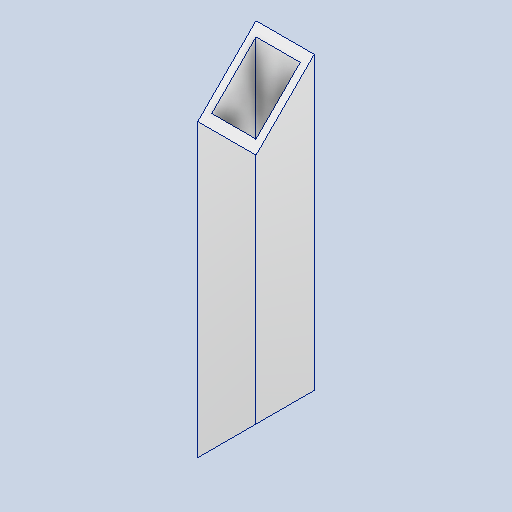
# Autodesk Inventor part: P407
Saved by Autodesk Inventor 2023 (Build 270158000, 158)
## iProperties
Created: 2022-08-29
Part Number: P407
Material: Aluminum 6061
Document SubType Name: Modeling
Designer: D.C. Eksteen
Density: 2.7 g/cm^3
Appearance: Aluminum - Flat
Author: D.C. Eksteen
Title: FRONT PLATFORM TUBE
Autodesk Inventor part; units mm, degrees
ref_plane "YZ Plane" through (0, 0, 0) normal (1, 0, 0) x (0, 1, 0)
ref_plane "XZ Plane" through (0, 0, 0) normal (0, 1, 0) x (-1, 0, 0)
ref_plane "XY Plane" through (0, 0, 0) normal (0, 0, 1) x (1, 0, 0)
sketch "Sketch1" plane through (0, 0, 0) normal (0, 1, 0) x (-1, 0, 0)
  line L0 (0, 0) -> (25, 0)
  line L1 (25, 0) -> (25, -25)
  line L2 (25, -25) -> (0, -25)
  line L3 (0, -25) -> (0, 0)
  line L4 (22, -22) -> (22, -3)
  line L5 (22, -3) -> (3, -3)
  line L6 (3, -3) -> (3, -22)
  line L7 (3, -22) -> (22, -22)
  dimension "d0" = 25
  dimension "d1" = 25
  dimension "d2" = 3
  constraints: 16 end point, 4 parallel, 2 perpendicular, 1 horizontal, 3 other
  measures "d0" distance of L1.end L2.end
  measures "d1" distance of L0.end L1.end
  measures "d2" distance between parallel lines of L1 L4
extrude "Extrusion1" add sketch "Sketch1" along normal blind 150
sketch "Sketch2" plane through (0, 0, 0) normal (1, 0, 0) x (0, 0, -1)
  line L0 (0, 0) -> (25, 0) projected
  line L1 (25, 0) -> (25, 150) projected
  line L2 (0, 150) -> (25, 150) projected
  line L3 (0, 0) -> (0, 150) projected
  line L4 (0, 0) -> (0, 150) projected
  line L5 (0, 150) -> (35.3553, 150) construction
  line L6 (25, 150) -> (0, 125)
  point P0 (25, 125)
  dimension "d14" = 45
  constraints: 4 end point, 2 point on line, 1 horizontal
  measures "d14" angle of L2 L6
extrude "Extrusion2" cut sketch "Sketch2" against normal blind 80 contours L3 L2 L6
sketch "Sketch3" plane through (0, 0, -25) normal (0, 0, -1) x (-1, 0, 0)
  line L0 (25, 125) -> (0, 125) projected
  line L1 (0, 0) -> (0, 125) projected
  line L2 (0, 0) -> (25, 0) projected
  line L3 (25, 0) -> (25, 125) projected
  line L4 (25, 0) -> (0, 25)
  dimension "d11" = 45
  constraints: 2 end point, 1 point on line
  measures "d11" angle of L2 L4
extrude "Extrusion3" cut sketch "Sketch3" against normal blind 100 contours L2 L1 L4
body "Solid1"
